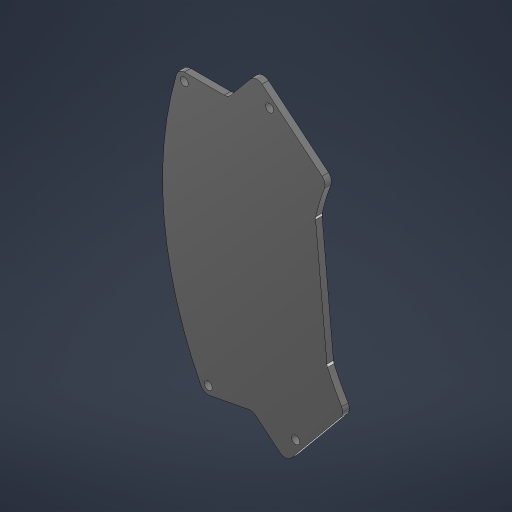
# Autodesk Inventor part: MainMCU_PCB
Saved by Autodesk Inventor 2024.2 (Build 282272000, 272)
## iProperties
Created: 2023-12-21
Part Number: MainMCU_PCB
Material: 一般
Document SubType Name: Modeling
Designer: Hanaoka
Density: 1 g/cm^3
Appearance: 既定
Author: Hanaoka
Autodesk Inventor part; units mm, degrees
ref_plane "YZ Plane" through (0, 0, 0) normal (1, 0, 0) x (0, 1, 0)
ref_plane "XZ Plane" through (0, 0, 0) normal (0, 1, 0) x (-1, 0, 0)
ref_plane "XY Plane" through (0, 0, 0) normal (0, 0, 1) x (1, 0, 0)
sketch "スケッチ1" plane through (0, 0, 0) normal (0, 0, 1) x (1, 0, 0)
  circle A0 centre (21.005288, 4.842186) radius 2
  circle A1 centre (0, 0) radius 2
  circle A2 centre (81.171801, -23.481667) radius 63
  arc A3 (-1.921226, 0.555779) -> (4.088443, -62.729672) centre (81.171801, -23.481667) ccw
  line L0 (0, 2) -> (9.827028, 2)
  line L1 (11.368602, 2.725814) -> (16.319283, 8.715397)
  line L2 (19.135043, 8.982785) -> (33.924305, -3.241258)
  line L3 (8.206239, 4.393532) -> (1.777293, 9.707368)
  line L4 (40.328272, 40.117124) -> (11.021999, 4.660921)
  arc A4 (9.827028, 2) -> (11.368602, 2.725814) centre (9.827028, 4) ccw
  arc A5 (19.135043, 8.982785) -> (16.319283, 8.715397) centre (17.860857, 7.441211) ccw
  arc A6 (34.516338, -5.502018) -> (38.734488, -49.921682) centre (81.171801, -23.481667) ccw
  circle A7 centre (5.870717, -61.822204) radius 2
  circle A8 centre (27.411976, -62.624114) radius 2
  line L5 (81.171801, -23.481667) -> (18.171801, -23.481667) construction
  line L6 (38.578569, -52.253469) -> (26.354526, -67.042731)
  line L7 (17.573011, -64.325196) -> (53.029214, -93.631469)
  line L8 (17.573011, -64.325196) -> (53.029214, -93.631469)
  line L9 (9.443415, -71.02153) -> (14.757251, -64.592584)
  line L10 (23.538766, -67.310119) -> (17.549183, -62.359438)
  arc A9 (23.538766, -67.310119) -> (26.354526, -67.042731) centre (24.812952, -65.768545) ccw
  line L11 (15.898547, -61.93676) -> (6.247168, -63.786456)
  arc A10 (17.549183, -62.359438) -> (15.898547, -61.93676) centre (16.274997, -63.901012) ccw
  arc A11 (34.516338, -5.502018) -> (33.924305, -3.241258) centre (32.65012, -4.782832) ccw
  arc A12 (38.578569, -52.253469) -> (38.734488, -49.921682) centre (37.036995, -50.979283) ccw
  circle A13 centre (5.870717, -61.822204) radius 1
  circle A14 centre (27.411976, -62.624114) radius 1
  circle A15 centre (21.005288, 4.842186) radius 1
  circle A16 centre (0, 0) radius 1
  line L12 (0, 0) -> (5.870717, -61.822204) construction
  line L13 (32.285214, -12.988736) -> (35.134053, -42.988736)
  point P0 (0, 0)
  point P1 (35.050768, -4.172335)
  point P2 (39.509645, -51.127006)
  dimension "d0" = 1.5
  dimension "d1" = 2
  dimension "d3" = 50
  dimension "d8" = 2
  dimension "d9" = 2
  dimension "d12" = 30
  constraints: 24 point on circle, 18 end point, 17 tangent, 12 centre point, 7 equal radius, 6 coincident, 4 parallel, 3 perpendicular, 2 horizontal, 2 point on line, 1 horizontal alignment, 1 other
  measures "d0" distance between parallel lines of L1 L4
  measures "d1" radius of A4
  measures "d3" radius of A6
  measures "d8" radius of A11
  measures "d9" diameter of A13
  measures "d12" vertical distance of L13.start L13.end
extrude "押し出し1" add sketch "スケッチ1" along normal blind 1.6 contours A0 | A8 | L2 A2 L6 A9 L10 A10 L11 A7 A3 A1 L0 A4 L1 A5 | L2 A11 A6 A12 L6 A2 | L13 A6 | A1 | A7
fillet "フィレット1" radius 2 2 edges at (35.1341, -42.9887, 0.8) (32.2852, -12.9887, 0.8)
